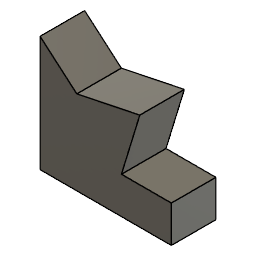
replay (Autodesk Fusion 360 design; units mm, degrees)
Autodesk Fusion 360 part; units mm, degrees
sketch "草图1" plane through (0, 0, 0) normal (0, 0, 1) x (1, 0, 0)
  line L0 (36, 9) -> (36, 23)
  line L1 (36, 23) -> (17, 23)
  line L2 (17, 23) -> (24, 46)
  line L3 (24, 46) -> (0, 41)
  line L4 (0, 41) -> (-14, 53)
  line L5 (-14, 53) -> (-14, 9)
  line L6 (-14, 9) -> (36, 9)
extrude "拉伸1" add sketch "草图1" along normal blind 17
